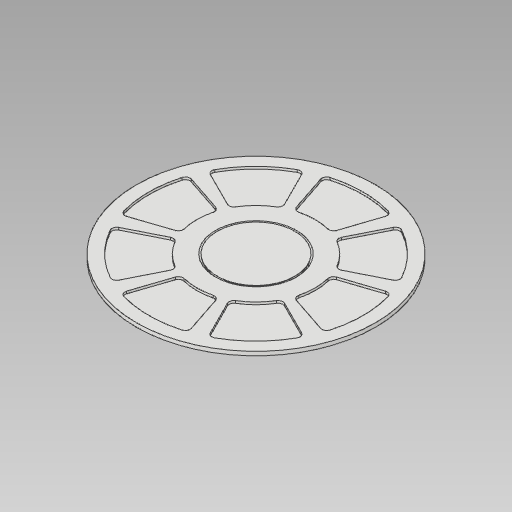
# Autodesk Inventor part: centre
Saved by Autodesk Inventor 2019.3 (Build 233278000, 278)
## iProperties
Created: 2019-03-01
Part Number: centre
Material: ABS Plastic
Document SubType Name: Modeling
Designer: WW
Density: 1.06 g/cm^3
Appearance: Smooth - White
Author: WW
Autodesk Inventor part; units mm, degrees
ref_plane "YZ Plane" through (0, 0, 0) normal (1, 0, 0) x (0, 1, 0)
ref_plane "XZ Plane" through (0, 0, 0) normal (0, 1, 0) x (-1, 0, 0)
ref_plane "XY Plane" through (0, 0, 0) normal (0, 0, 1) x (1, 0, 0)
sketch "Sketch1" plane through (0, 0, 0) normal (0, 0, 1) x (1, 0, 0)
  line L0 (0, 0) -> (0, -126.8557)
  line L1 (0, 0) -> (25, 0)
  line L2 (25, 0) -> (23.75, 1.25)
  line L3 (23.75, 1.25) -> (25, 2.5)
  line L4 (25, 2.5) -> (0, 2.5)
  line L5 (0, 2.5) -> (0, 0)
  line L6 (25.9899, 2.5) -> (24.7399, 1.25)
  line L7 (24.7399, 1.25) -> (25.9899, 0)
  line L8 (25.9899, 0) -> (76.75, 0)
  line L9 (76.75, 0) -> (76.75, 2.5)
  line L10 (76.75, 2.5) -> (25.9899, 2.5)
  point P0 (0, 1.25)
  dimension "d0" = 45
  dimension "d1" = 153.5
  dimension "d2" = 2.5
  dimension "d3" = 0.7
  dimension "d4" = 50
  constraints: 22 end point, 5 perpendicular, 4 horizontal alignment, 3 horizontal, 1 midpoint, 1 parallel, 1 vertical
  measures "d0" angle of L1 L2
  measures "d1" diameter of L9 L0
  measures "d2" distance of L4.end L0.start
  measures "d3" distance between parallel lines of L6 L3
  measures "d4" diameter of L3.end L0
revolve "Revolution1" add sketch "Sketch1" angle 360 about axis through (0, 0, 0) along (0, -1, 0)
sketch "Sketch2" plane through (0, 2.5, 0) normal (0, 1, 0) x (1, 0, 0)
  circle A0 centre (0, 0) radius 25.9899 projected
  circle A1 centre (0, 0) radius 76.75 projected
  circle A2 centre (0, 0) radius 68.75
  circle A3 centre (0, 0) radius 37.9899
  line L0 (-21.7163, 65.2301) -> (-12, 36.0449)
  line L1 (12, 36.0449) -> (21.7163, 65.2301)
  line L2 (-12, 36.0449) -> (12, 36.0449) construction
  line L3 (-61.4804, 30.7689) -> (-33.9729, 17.0023)
  line L4 (-17.0023, 33.9729) -> (-30.7689, 61.4804)
  line L5 (-65.2301, -21.7163) -> (-36.0449, -12)
  line L6 (-36.0449, 12) -> (-65.2301, 21.7163)
  line L7 (-30.7689, -61.4804) -> (-17.0023, -33.9729)
  line L8 (-33.9729, -17.0023) -> (-61.4804, -30.7689)
  line L9 (21.7163, -65.2301) -> (12, -36.0449)
  line L10 (-12, -36.0449) -> (-21.7163, -65.2301)
  line L11 (61.4804, -30.7689) -> (33.9729, -17.0023)
  line L12 (17.0023, -33.9729) -> (30.7689, -61.4804)
  line L13 (65.2301, 21.7163) -> (36.0449, 12)
  line L14 (36.0449, -12) -> (65.2301, -21.7163)
  line L15 (30.7689, 61.4804) -> (17.0023, 33.9729)
  line L16 (33.9729, 17.0023) -> (61.4804, 30.7689)
  dimension "d6" = 8
  dimension "d7" = 12
  dimension "d10" = 360
  dimension "d12" = 24
  constraints: 34 end point, 4 point on circle, 2 centre point, 2 line through centre, 1 horizontal, 49 other
  measures "d6" radial gap between concentric circles of A1 A2
  measures "d7" radial gap between concentric circles of A0 A3
  measures "d12" distance of L0.end L1.start
extrude "Extrusion1" cut sketch "Sketch2" against normal blind 1.5 contours L1 A3 L0 A2
fillet "Fillet1" radius 3 4 edges at (12, 1.75, -36.0449) (21.7163, 1.75, -65.2301) (-12, 1.75, -36.0449) (-21.7163, 1.75, -65.2301)
pattern_circular "Circular Pattern1" count 8 over 360 about axis through (0, 1.25, 0) along (0, -1, 0) of "Extrusion1", "Fillet1"
body "Solid1"
